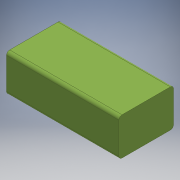
# Autodesk Inventor part: Li-Pol
Saved by Autodesk Inventor 2018 (Build 220112000, 112)
## iProperties
Created: 2018-08-13
Part Number: Li-Pol
Material: Ogólny
Document SubType Name: Modeling
Designer: Wojciech
Density: 1.87605 g/cm^3
Appearance: Oliwkowozielona
Mass: 113 g
Surface Area: 99.2191 cm^2
Volume: 60.2328 cm^3
Author: Wojciech
Autodesk Inventor part; units mm, degrees
ref_plane "YZ Plane" through (0, 0, 0) normal (1, 0, 0) x (0, 1, 0)
ref_plane "XZ Plane" through (0, 0, 0) normal (0, 1, 0) x (-1, 0, 0)
ref_plane "XY Plane" through (0, 0, 0) normal (0, 0, 1) x (1, 0, 0)
sketch "Szkic1" plane through (0, 0, 0) normal (0, 0, 1) x (1, 0, 0)
  line L0 (-36, -17.5) -> (36, -17.5)
  line L1 (36, -17.5) -> (36, 17.5)
  line L2 (36, 17.5) -> (-36, 17.5)
  line L3 (-36, 17.5) -> (-36, -17.5)
  line L4 (-36, -17.5) -> (36, 17.5) construction
  line L5 (36, -17.5) -> (-36, 17.5) construction
  point P0 (0, 0)
  dimension "d0" = 72
  dimension "d1" = 35
  constraints: 12 end point, 2 midpoint, 2 parallel, 1 horizontal, 1 perpendicular
  measures "d0" distance of L2.end L1.end
  measures "d1" distance of L1.end L0.end
extrude "Wyciągnięcie proste1" add sketch "Szkic1" along normal blind 24
fillet "Zaokrąglenie1" radius 2 4 edges at (0, 17.5, 0) (0, -17.5, 0) (0, -17.5, 24) (0, 17.5, 24)
